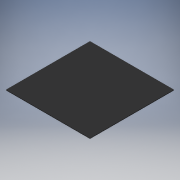
# Autodesk Inventor part: silicone heater
Saved by Autodesk Inventor 2017 (Build 210142000, 142)
## iProperties
Part Number: silicone heater
Material: Kautschuk
Document SubType Name: Modeling
Designer: Till
Density: 0.93 g/cm^3
Appearance: Gummi - schwarz
Author: Till
Autodesk Inventor part; units mm, degrees
ref_plane "YZ Plane" through (0, 0, 0) normal (1, 0, 0) x (0, 1, 0)
ref_plane "XZ Plane" through (0, 0, 0) normal (0, 1, 0) x (-1, 0, 0)
ref_plane "XY Plane" through (0, 0, 0) normal (0, 0, 1) x (1, 0, 0)
sketch "Skizze1" plane through (0, 0, 0) normal (0, 0, 1) x (1, 0, 0)
  line L0 (-148, -150) -> (148, -150)
  line L1 (150, -148) -> (150, 148)
  line L2 (148, 150) -> (-148, 150)
  line L3 (-150, 148) -> (-150, -148)
  line L4 (-150, -150) -> (150, 150) construction
  line L5 (150, -150) -> (-150, 150) construction
  arc A0 (-148, 150) -> (-150, 148) centre (-148, 148) ccw
  arc A1 (150, 148) -> (148, 150) centre (148, 148) ccw
  arc A2 (148, -150) -> (150, -148) centre (148, -148) ccw
  arc A3 (-150, -148) -> (-148, -150) centre (-148, -148) ccw
  point P0 (0, 0)
  dimension "d0" = 300
  dimension "d1" = 300
  dimension "d4" = 2
  constraints: 12 end point, 8 point on circle, 8 point on line, 8 tangent, 4 centre point, 3 equal radius, 2 midpoint, 2 parallel, 1 horizontal, 1 perpendicular
  measures "d0" distance of L5.end L4.end
  measures "d1" distance of L4.end L5.start
  measures "d4" radius of A0
extrude "Extrusion1" add sketch "Skizze1" along normal blind 2
